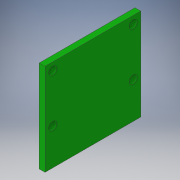
# Autodesk Inventor part: Booard
Saved by Autodesk Inventor 2018 (Build 220112000, 112)
## iProperties
Created: 2018-05-02
Part Number: Booard
Material: Generic
Document SubType Name: Modeling
Designer: Ajith Thomas
Density: 1 g/cm^3
Appearance: Default
Author: Ajith Thomas
Autodesk Inventor part; units mm, degrees
ref_plane "YZ Plane" through (0, 0, 0) normal (1, 0, 0) x (0, 1, 0)
ref_plane "XZ Plane" through (0, 0, 0) normal (0, 1, 0) x (-1, 0, 0)
ref_plane "XY Plane" through (0, 0, 0) normal (0, 0, 1) x (1, 0, 0)
sketch "Sketch1" plane through (0, 0, 0) normal (1, 0, 0) x (0, 1, 0)
  line L0 (12, 12.5) -> (-12, 12.5)
  line L1 (-12, 12.5) -> (-12, -12.5)
  line L2 (-12, -12.5) -> (12, -12.5)
  line L3 (12, -12.5) -> (12, 12.5)
  line L4 (12, 12.5) -> (-12, -12.5) construction
  line L5 (-12, 12.5) -> (12, -12.5) construction
  circle A0 centre (10, 10.5) radius 1.05
  line L6 (12, 0) -> (-12, 0) construction
  circle A1 centre (-2.5, 10.5) radius 1.05
  circle A2 centre (10, -10.5) radius 1.05
  circle A3 centre (-2.5, -10.5) radius 1.05
  point P0 (0, 0)
  dimension "d0" = 24
  dimension "d1" = 25
  dimension "d2" = 2.1
  dimension "d3" = 2
  dimension "d4" = 2
  dimension "d5" = 2.1
  dimension "d6" = 12.5
  dimension "d7" = 2
  constraints: 14 end point, 4 centre point, 4 midpoint, 2 parallel, 2 symmetric about line, 1 horizontal, 1 perpendicular, 2 other
  measures "d0" distance of L2.end L1.end
  measures "d1" distance of L1.end L0.end
  measures "d2" diameter of A0
  measures "d3" distance from line of L3 A0.centre
  measures "d4" distance from line of L0 A0.centre
  measures "d5" diameter of A1
  measures "d6" distance of A0.centre A1.centre
  measures "d7" distance from line of L0 A1.centre
extrude "Extrusion1" add sketch "Sketch1" along normal mid plane 1.5
body "Solid1"
